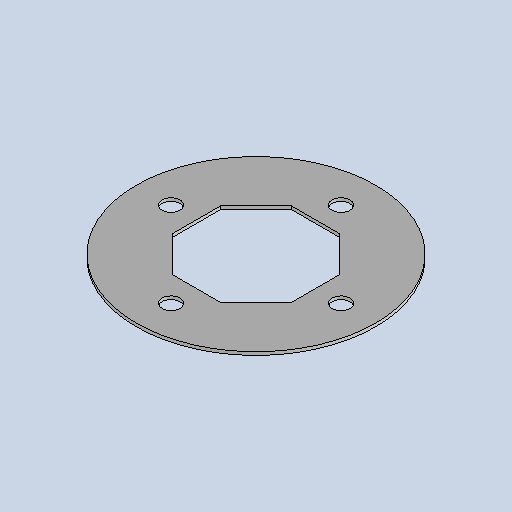
# Autodesk Inventor part: TZS 0972 funnel FLANGE 50-90
Saved by Autodesk Inventor 2025.3 (Build 293356030, 356C)
## iProperties
Created: 2025-06-24
Part Number: TZS 0972 funnel FLANGE 50-90
Material: Stainless Steel
Description: DIE16(5)|\ 90°|corrY -___°|X_____|bom___
Document SubType Name: Sheet Metal
Designer: user
Mass: 683.685 g
Surface Area: 608.472 cm^2
Volume: 85.4606 cm^3
Density: 8 g/cm^3
Flat Pattern Width: 22.5 cm
Flat Pattern Length: 22.5 cm
Flat Pattern Area: 506.25 cm^2
Sheet Metal Rule: Default
Sheet Metal Width: 225,000 mm
Sheet Metal Length: 225,000 mm
Sheet Metal Area: 50625,000 mm^2
Appearance: Default
Author: user
Autodesk Inventor part; units mm, degrees
ref_plane "YZ Plane" through (0, 0, 0) normal (1, 0, 0) x (0, 1, 0)
ref_plane "XZ Plane" through (0, 0, 0) normal (0, 1, 0) x (-1, 0, 0)
ref_plane "XY Plane" through (0, 0, 0) normal (0, 0, 1) x (1, 0, 0)
sketch "Sketch1" plane through (0, 0, 0) normal (0, 0, 1) x (1, 0, 0)
  circle A0 centre (0, 0) radius 112.5
  line L0 (56, 56) -> (-56, 56)
  line L1 (-56, 56) -> (-56, -56)
  line L2 (-56, -56) -> (56, -56)
  line L3 (56, -56) -> (56, 56)
  line L4 (56, 56) -> (-56, -56) construction
  line L5 (-56, 56) -> (56, -56) construction
  dimension "d157" = 225
  dimension "d158" = 112
  dimension "d159" = 112
  measures "d157" diameter of A0
  measures "d158" distance of L2.end L1.end
  measures "d159" distance of L1.end L0.end
extrude "Plate5" add sketch "Sketch1" along normal blind 3
sketch "Sketch7" plane through (0, 0, 0) normal (0, 0, -1) x (-1, 0, 0)
  circle A0 centre (0, 80) radius 8.5
  point P0 (0, 0)
  dimension "d160" = 17
  dimension "d161" = 80
  constraints: 1 centre point, 1 vertical alignment
  measures "d160" diameter of A0
  measures "d161" distance of point (0, 0) A0.centre
extrude "Cut1" cut sketch "Sketch7" against normal blind 3
pattern_circular "Circular Pattern1" count 4 over 360 about axis through (0, 0, -10) along (0, 0, 1) of "Cut1"
chamfer "Corner Chamfer2" distance 33 angle 45 4 edges at (-56, -56, 1.5) (56, -56, 1.5) (-56, 56, 1.5) (56, 56, 1.5)
body "Solid3"
